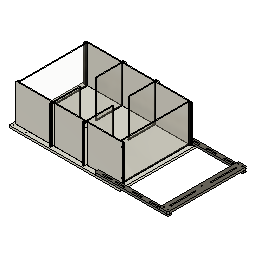
3ChamberBox (Autodesk Fusion 360 design; units mm, degrees)
Autodesk Fusion 360 part; units mm, degrees
sketch "Base" plane through (0, 0, 0) normal (0, 0, 1) x (1, 0, 0)
  line L0 (0, 0) -> (660.4, 0)
  line L1 (660.4, 0) -> (660.4, 469.9)
  line L2 (660.4, 469.9) -> (0, 469.9)
  line L3 (0, 469.9) -> (0, 0)
  line L4 (636.651, 437.261) -> (636.651, 32.639)
  line L5 (23.749, 32.639) -> (23.749, 437.261)
  line L6 (30.226, 32.639) -> (30.226, 437.261)
  line L7 (630.174, 437.261) -> (630.174, 32.639)
  line L8 (233.4895, 459.4352) -> (233.4895, 459.4352)
  line L9 (233.4895, 10.4648) -> (233.4895, 10.4648)
  line L10 (429.1965, 459.4352) -> (429.1965, 459.4352)
  line L11 (429.1965, 10.4648) -> (429.1965, 10.4648)
  line L12 (23.749, 437.261) -> (11.4935, 437.261)
  line L13 (8.255, 440.4995) -> (8.255, 440.4995)
  line L14 (11.4935, 443.738) -> (23.749, 443.738)
  line L15 (636.651, 437.261) -> (648.9065, 437.261)
  line L16 (652.145, 440.4995) -> (652.145, 440.4995)
  line L17 (648.9065, 443.738) -> (636.651, 443.738)
  line L18 (636.651, 26.162) -> (648.9065, 26.162)
  line L19 (652.145, 29.4005) -> (652.145, 29.4005)
  line L20 (648.9065, 32.639) -> (636.651, 32.639)
  line L21 (432.435, 13.7033) -> (432.435, 26.162)
  line L22 (432.435, 32.639) -> (432.435, 190.4057)
  line L23 (425.958, 190.4057) -> (425.958, 32.639)
  line L24 (425.958, 26.162) -> (425.958, 13.7033)
  line L25 (630.174, 32.639) -> (432.435, 32.639)
  line L26 (636.651, 26.162) -> (432.435, 26.162)
  line L27 (425.958, 32.639) -> (236.728, 32.639)
  line L28 (230.251, 32.639) -> (30.226, 32.639)
  line L29 (230.251, 13.7033) -> (230.251, 26.162)
  line L30 (230.251, 32.639) -> (230.251, 190.4057)
  line L31 (236.728, 190.4057) -> (236.728, 32.639)
  line L32 (236.728, 26.162) -> (236.728, 13.7033)
  line L33 (425.958, 26.162) -> (236.728, 26.162)
  line L34 (230.251, 26.162) -> (23.749, 26.162)
  line L35 (23.749, 443.738) -> (230.251, 443.738)
  line L36 (230.251, 282.6512) -> (230.251, 437.261)
  line L37 (230.251, 443.738) -> (230.251, 456.1967)
  line L38 (30.226, 437.261) -> (230.251, 437.261)
  line L39 (236.728, 456.1967) -> (236.728, 443.738)
  line L40 (236.728, 437.261) -> (236.728, 282.6512)
  line L41 (236.728, 443.738) -> (425.958, 443.738)
  line L42 (432.435, 443.738) -> (636.651, 443.738)
  line L43 (425.958, 456.1967) -> (425.958, 443.738)
  line L44 (425.958, 437.261) -> (425.958, 282.6512)
  line L45 (432.435, 282.6512) -> (432.435, 437.261)
  line L46 (432.435, 443.738) -> (432.435, 456.1967)
  line L47 (236.728, 437.261) -> (425.958, 437.261)
  line L48 (432.435, 437.261) -> (630.174, 437.261)
  line L49 (23.749, 26.162) -> (11.4935, 26.162)
  line L50 (8.255, 29.4005) -> (8.255, 29.4005)
  line L51 (11.4935, 32.639) -> (23.749, 32.639)
  arc A0 (8.255, 440.4995) -> (11.4935, 437.261) centre (11.4935, 440.4995) ccw
  arc A1 (11.4935, 443.738) -> (8.255, 440.4995) centre (11.4935, 440.4995) ccw
  arc A2 (233.4895, 459.4352) -> (230.251, 456.1967) centre (233.4895, 456.1967) ccw
  arc A3 (236.728, 456.1967) -> (233.4895, 459.4352) centre (233.4895, 456.1967) ccw
  arc A4 (429.1965, 459.4352) -> (425.958, 456.1967) centre (429.1965, 456.1967) ccw
  arc A5 (432.435, 456.1967) -> (429.1965, 459.4352) centre (429.1965, 456.1967) ccw
  arc A6 (652.145, 440.4995) -> (648.9065, 443.738) centre (648.9065, 440.4995) ccw
  arc A7 (648.9065, 437.261) -> (652.145, 440.4995) centre (648.9065, 440.4995) ccw
  arc A8 (652.145, 29.4005) -> (648.9065, 32.639) centre (648.9065, 29.4005) ccw
  arc A9 (648.9065, 26.162) -> (652.145, 29.4005) centre (648.9065, 29.4005) ccw
  arc A10 (429.1965, 10.4648) -> (432.435, 13.7033) centre (429.1965, 13.7033) ccw
  arc A11 (425.958, 13.7033) -> (429.1965, 10.4648) centre (429.1965, 13.7033) ccw
  arc A12 (230.251, 13.7033) -> (233.4895, 10.4648) centre (233.4895, 13.7033) ccw
  arc A13 (233.4895, 10.4648) -> (236.728, 13.7033) centre (233.4895, 13.7033) ccw
  arc A14 (8.255, 29.4005) -> (11.4935, 26.162) centre (11.4935, 29.4005) ccw
  arc A15 (11.4935, 32.639) -> (8.255, 29.4005) centre (11.4935, 29.4005) ccw
  line L52 (230.8352, 283.2354) -> (236.1438, 283.2354)
  line L53 (236.1438, 437.8452) -> (426.5422, 437.8452)
  line L54 (426.5422, 283.2354) -> (431.8508, 283.2354)
  line L55 (431.8508, 283.2354) -> (431.8508, 455.8538)
  line L56 (630.7582, 437.8452) -> (630.7582, 32.0548)
  line L57 (431.8508, 189.8215) -> (426.5422, 189.8215)
  line L58 (426.5422, 32.0548) -> (236.1438, 32.0548)
  line L59 (236.1438, 189.8215) -> (236.1438, 14.0462)
  line L60 (236.1438, 189.8215) -> (230.8352, 189.8215)
  line L61 (230.8352, 14.0462) -> (230.8352, 189.8215)
  line L62 (29.6418, 32.0548) -> (29.6418, 437.8452)
  line L63 (426.5422, 455.8538) -> (426.5422, 283.2354)
  line L64 (236.1438, 443.1538) -> (426.5422, 443.1538)
  line L65 (236.1438, 455.8538) -> (236.1438, 283.2354)
  line L66 (230.8352, 283.2354) -> (230.8352, 455.8538)
  line L67 (23.749, 443.1538) -> (230.8352, 443.1538)
  line L68 (11.6332, 443.1538) -> (23.749, 443.1538)
  line L69 (230.8352, 437.8452) -> (11.6332, 437.8452)
  line L70 (24.3332, 32.0548) -> (24.3332, 437.8452)
  line L71 (11.6332, 32.0548) -> (230.8352, 32.0548)
  line L72 (23.749, 26.7462) -> (11.6332, 26.7462)
  line L73 (230.8352, 26.7462) -> (23.749, 26.7462)
  line L74 (426.5422, 26.7462) -> (236.1438, 26.7462)
  line L75 (426.5422, 189.8215) -> (426.5422, 14.0462)
  line L76 (431.8508, 14.0462) -> (431.8508, 189.8215)
  line L77 (636.651, 26.7462) -> (431.8508, 26.7462)
  line L78 (636.651, 26.7462) -> (648.7668, 26.7462)
  line L79 (648.7668, 32.0548) -> (431.8508, 32.0548)
  line L80 (636.0668, 437.8452) -> (636.0668, 32.0548)
  line L81 (431.8508, 437.8452) -> (648.7668, 437.8452)
  line L82 (648.7668, 443.1538) -> (636.651, 443.1538)
  line L83 (431.8508, 443.1538) -> (636.651, 443.1538)
  line L84 (648.7668, 32.0548) -> (648.7668, 26.7462)
  line L85 (648.7668, 443.1538) -> (648.7668, 437.8452)
  line L86 (426.5422, 455.8538) -> (431.8508, 455.8538)
  line L87 (241.427, 455.8538) -> (230.8352, 455.8538)
  line L88 (11.6332, 437.8452) -> (11.6332, 443.1538)
  line L89 (11.6332, 32.0548) -> (11.6332, 26.7462)
  line L90 (230.8352, 14.0462) -> (236.1438, 14.0462)
  line L91 (421.259, 14.0462) -> (437.134, 14.0462)
  line L92 (437.134, 26.7462) -> (437.134, 14.0462)
  line L93 (421.259, 26.7462) -> (421.259, 14.0462)
  line L94 (241.427, 26.7462) -> (241.427, 14.0462)
  line L95 (241.427, 14.0462) -> (236.1438, 14.0462)
  line L96 (225.552, 26.7462) -> (225.552, 14.0462)
  line L97 (225.552, 14.0462) -> (230.8352, 14.0462)
  line L98 (11.6332, 32.0548) -> (11.6332, 37.338)
  line L99 (11.6332, 37.338) -> (24.3332, 37.338)
  line L100 (11.6332, 437.8452) -> (11.6332, 432.562)
  line L101 (11.6332, 432.562) -> (24.3332, 432.562)
  line L102 (225.552, 443.1538) -> (225.552, 455.8538)
  line L103 (225.552, 455.8538) -> (230.8352, 455.8538)
  line L104 (241.427, 443.1538) -> (241.427, 455.8538)
  line L105 (421.259, 443.1538) -> (421.259, 455.8538)
  line L106 (421.259, 455.8538) -> (426.5422, 455.8538)
  line L107 (437.134, 443.1538) -> (437.134, 455.8538)
  line L108 (437.134, 455.8538) -> (431.8508, 455.8538)
  line L109 (636.0668, 432.562) -> (648.7668, 432.562)
  line L110 (648.7668, 432.562) -> (648.7668, 437.8452)
  line L111 (636.0668, 37.338) -> (648.7668, 37.338)
  line L112 (648.7668, 37.338) -> (648.7668, 32.0548)
  circle A16 centre (12.7, 457.2) radius 2.5527
  circle A17 centre (88.9, 457.2) radius 2.5527
  circle A18 centre (12.7, 12.7) radius 2.5527
  circle A19 centre (88.9, 12.7) radius 2.5527
  circle A20 centre (647.7, 12.7) radius 2.5527
  circle A21 centre (571.5, 12.7) radius 2.5527
  circle A22 centre (647.7, 457.2) radius 2.5527
  circle A23 centre (571.5, 457.2) radius 2.5527
  arc A24 (236.728, 190.4057) -> (230.251, 190.4057) centre (233.4895, 190.4057) ccw
  arc A25 (230.251, 282.6512) -> (236.728, 282.6512) centre (233.4895, 282.6512) ccw
  arc A26 (425.958, 282.6512) -> (432.435, 282.6512) centre (429.1965, 282.6512) ccw
  arc A27 (432.435, 190.4057) -> (425.958, 190.4057) centre (429.1965, 190.4057) ccw
  dimension "d1" = 660.4
  dimension "d2" = 469.9
  dimension "d3" = 26.162
  dimension "d4" = 26.162
  dimension "d5" = 23.749
  dimension "d6" = 23.749
  dimension "d8" = 200.025
  dimension "d9" = 6.477
  dimension "d10" = 197.739
  dimension "d11" = 6.477
  dimension "d22" = 3.2385
  dimension "d30" = 12.7
  dimension "d31" = 12.7
  dimension "d33" = 12.7
  dimension "d34" = 5.2832
  dimension "d35" = 5.2832
  dimension "d36" = 5.2832
  dimension "d37" = 5.2832
  dimension "d38" = 12.7
  dimension "d39" = 12.7
  dimension "d40" = 12.7
  dimension "d41" = 12.7
  dimension "d42" = 5.2832
  dimension "d43" = 5.2832
  dimension "d44" = 12.7
  dimension "d45" = 12.7
  dimension "d46" = 12.7
  dimension "d47" = 190.3984
  dimension "d48" = 12.7
  dimension "d49" = 5.2832
  dimension "d50" = 5.2832
  dimension "d51" = 12.7
  dimension "d52" = 5.2832
  dimension "d53" = 12.7
  dimension "d54" = 12.7
  dimension "d55" = 5.2832
  dimension "d56" = 12.7
  dimension "d57" = 12.7
  dimension "d58" = 5.2832
  dimension "d59" = 12.7
  dimension "d60" = 5.2832
  dimension "d61" = 12.7
  dimension "d62" = 12.7
  dimension "d63" = 12.7
  dimension "d195" = 5.1054
  dimension "d196" = 5.1054
  dimension "d197" = 12.7
  dimension "d198" = 88.9
  dimension "d199" = 12.7
  dimension "d200" = 12.7
  dimension "d201" = 5.1054
  dimension "d202" = 5.1054
  dimension "d203" = 12.7
  dimension "d204" = 88.9
  dimension "d205" = 12.7
  dimension "d206" = 12.7
  dimension "d207" = 5.1054
  dimension "d208" = 5.1054
  dimension "d209" = 12.7
  dimension "d210" = 88.9
  dimension "d211" = 12.7
  dimension "d212" = 12.7
  dimension "d213" = 5.1054
  dimension "d214" = 5.1054
  dimension "d215" = 12.7
  dimension "d216" = 88.9
  dimension "d217" = 12.7
  dimension "d218" = 12.7
  constraint horizontal L0
  constraint vertical L1
  constraint horizontal L2
  constraint vertical L3
  constraint coincident L0.start L3.end
  constraint horizontal L35
  constraint vertical L4
  constraint horizontal L26
  constraint vertical L5
  constraint vertical L39
  constraint vertical L29
  constraint vertical L43
  constraint vertical L21
  constraint coincident L36.start L29
  constraint collinear L29 L36
  constraint collinear L31 L39
  constraint coincident L23.start L43
  constraint collinear L21 L45
  constraint collinear L23 L43
  constraint perpendicular L5 L12
  constraint perpendicular L5 L14
  constraint parallel L25 L26
  constraint parallel L5 L6
  constraint parallel L35 L38
  constraint parallel L4 L7
  constraint perpendicular L4 L15
  constraint perpendicular L4 L17
  constraint perpendicular L7 L18
  constraint perpendicular L4 L20
  constraint collinear L21 L22
  constraint coincident L23.end L25
  constraint coincident L24.start L26
  constraint collinear L23 L24
  constraint collinear L25 L27
  constraint collinear L26 L33
  constraint coincident L28.start L29
  constraint collinear L27 L28
  constraint coincident L29.end L33
  constraint collinear L29 L30
  constraint collinear L31 L32
  constraint collinear L33 L34
  constraint coincident L35.end L36
  constraint collinear L35 L41
  constraint collinear L36 L37
  constraint coincident L40.start L39
  constraint collinear L38 L47
  constraint collinear L39 L40
  constraint coincident L42.start L45
  constraint collinear L41 L42
  constraint collinear L43 L44
  constraint coincident L45.end L47
  constraint collinear L45 L46
  constraint collinear L47 L48
  constraint perpendicular L5 L49
  constraint perpendicular L5 L51
  constraint tangent L12 A0
  constraint tangent L14 A1
  constraint equal A0 A1
  constraint tangent L37 A2
  constraint equal A0 A2
  constraint tangent L39 A3
  constraint equal A0 A3
  constraint tangent L43 A4
  constraint equal A0 A4
  constraint tangent L46 A5
  constraint equal A0 A5
  constraint tangent L17 A6
  constraint equal A0 A6
  constraint tangent L15 A7
  constraint equal A0 A7
  constraint tangent L20 A8
  constraint equal A0 A8
  constraint tangent L18 A9
  constraint equal A0 A9
  constraint tangent L21 A10
  constraint equal A0 A10
  constraint tangent L24 A11
  constraint equal A0 A11
  constraint tangent L29 A12
  constraint equal A0 A12
  constraint tangent L32 A13
  constraint equal A0 A13
  constraint tangent L49 A14
  constraint equal A0 A14
  constraint tangent L51 A15
  constraint equal A0 A15
  constraint parallel L43 L63
  constraint parallel L41 L64
  constraint parallel L39 L65
  constraint parallel L37 L66
  constraint parallel L35 L67
  constraint parallel L14 L68
  constraint parallel L12 L69
  constraint parallel L5 L70
  constraint parallel L51 L71
  constraint parallel L49 L72
  constraint parallel L34 L73
  constraint parallel L29 L61
  constraint parallel L32 L59
  constraint parallel L33 L74
  constraint parallel L24 L75
  constraint parallel L21 L76
  constraint parallel L26 L77
  constraint parallel L18 L78
  constraint parallel L20 L79
  constraint parallel L4 L80
  constraint parallel L15 L81
  constraint parallel L17 L82
  constraint parallel L42 L83
  constraint parallel L46 L55
  constraint coincident L67.end L66
  constraint parallel L40 L65
  constraint parallel L47 L53
  constraint parallel L44 L63
  constraint parallel L45 L55
  constraint parallel L48 L81
  constraint parallel L7 L56
  constraint parallel L25 L79
  constraint parallel L22 L76
  constraint parallel L23 L75
  constraint parallel L27 L58
  constraint parallel L31 L59
  constraint parallel L30 L61
  constraint parallel L28 L71
  constraint parallel L6 L62
  constraint parallel L38 L69
  constraint parallel L36 L66
  constraint coincident L64.start L65
  constraint coincident L64.end L63
  constraint coincident L81.start L55
  constraint coincident L77.end L76
  constraint coincident L74.start L75
  constraint coincident L71.end L61
  constraint coincident L58.end L59
  constraint perpendicular L78 L84
  constraint perpendicular L82 L85
  constraint perpendicular L55 L86
  constraint perpendicular L65 L87
  constraint perpendicular L68 L88
  constraint perpendicular L72 L89
  constraint perpendicular L61 L90
  constraint perpendicular L76 L91
  constraint coincident L77 L92.start
  constraint perpendicular L26 L92
  constraint perpendicular L21 L91
  constraint coincident L74 L93.start
  constraint perpendicular L33 L93
  constraint perpendicular L24 L91
  constraint coincident L74 L94.start
  constraint perpendicular L33 L94
  constraint coincident L59 L90.end
  constraint perpendicular L59 L95
  constraint coincident L73 L96.start
  constraint perpendicular L34 L96
  constraint coincident L61 L90.start
  constraint perpendicular L61 L97
  constraint coincident L71 L89.start
  constraint perpendicular L51 L98
  constraint coincident L70 L99.end
  constraint perpendicular L70 L99
  constraint coincident L69 L88.start
  constraint perpendicular L12 L100
  constraint coincident L70 L101.end
  constraint perpendicular L70 L101
  constraint coincident L67 L102.start
  constraint perpendicular L67 L102
  constraint coincident L66 L87.end
  constraint perpendicular L66 L103
  constraint coincident L64 L104.start
  constraint perpendicular L41 L104
  constraint perpendicular L39 L87
  constraint coincident L64 L105.start
  constraint perpendicular L64 L105
  constraint coincident L63 L86.start
  constraint perpendicular L63 L106
  constraint coincident L83 L107.start
  constraint perpendicular L42 L107
  constraint coincident L55 L86.end
  constraint perpendicular L55 L108
  constraint coincident L80 L109.start
  constraint perpendicular L80 L109
  constraint coincident L81 L85.end
  constraint perpendicular L81 L110
  constraint coincident L80 L111.start
  constraint perpendicular L80 L111
  constraint coincident L79 L84.start
  constraint perpendicular L79 L112
  constraint tangent L40 A25
  constraint tangent L31 A24
  constraint tangent L45 A26
  constraint tangent L22 A27
  measures "d1" distance of L0.start L0.end
  measures "d2" distance of L0.start L2.end
  measures "d3" distance of L2 L35
  measures "d4" distance of L0 L26
  measures "d5" distance of L3 L5
  measures "d6" distance of L1 L4
  measures "d8" distance of L6 L29
  measures "d9" distance of L29 L39
  measures "d10" distance of L7 L21
  measures "d11" distance of L21 L43
  measures "d22" radius of A0
  measures "d30" distance of L77 L91
  measures "d31" distance of L74 L91
  measures "d33" distance of L74 L91
  measures "d34" distance of L76 L92
  measures "d35" distance of L75 L93
  measures "d36" distance of L61 L96
  measures "d37" distance of L59 L94
  measures "d38" distance of L73 L97
  measures "d39" distance of L73 L90
  measures "d40" distance of L74 L95
  measures "d41" distance of L70 L98
  measures "d42" distance of L71 L99
  measures "d43" distance of L69 L101
  measures "d44" distance of L70 L100
  measures "d45" distance of L67 L103
  measures "d46" distance of L67 L87
  measures "d47" distance of L64.end L64.start
  measures "d48" distance of L64 L87
  measures "d49" distance of L65 L104
  measures "d50" distance of L66 L102
  measures "d51" distance of L64 L106
  measures "d52" distance of L63 L105
  measures "d53" distance of L64 L86
  measures "d54" distance of L83 L108
  measures "d55" distance of L55 L107
  measures "d56" distance of L80 L110
  measures "d57" distance of L80 L85
  measures "d58" distance of L81 L109
  measures "d59" distance of L80 L112
  measures "d60" distance of L79 L111
  measures "d61" distance of L80 L84
  measures "d62" distance of L70 L88
  measures "d63" distance of L70 L89
  measures "d195" diameter of A16
  measures "d196" diameter of A17
  measures "d197" distance of L3 A16.centre
  measures "d198" distance of L3 A17.centre
  measures "d199" distance of L2 A16.centre
  measures "d200" distance of L2 A17.centre
  measures "d201" diameter of A18
  measures "d202" diameter of A19
  measures "d203" distance of L3 A18.centre
  measures "d204" distance of L3 A19.centre
  measures "d205" distance of L0 A18.centre
  measures "d206" distance of L0 A19.centre
  measures "d207" diameter of A20
  measures "d208" diameter of A21
  measures "d209" distance of L1 A20.centre
  measures "d210" distance of L1 A21.centre
  measures "d211" distance of L0 A20.centre
  measures "d212" distance of L0 A21.centre
  measures "d213" diameter of A22
  measures "d214" diameter of A23
  measures "d215" distance of L1 A22.centre
  measures "d216" distance of L1 A23.centre
  measures "d217" distance of L2 A22.centre
  measures "d218" distance of L2 A23.centre
extrude "Extrude1" add sketch "Base" against normal blind 12.7 contours L0 L1 L2 L3 | L4 L15 L109 L110 | L4 L15 L80 L81 L109 L110 | L4 L80 L109 L111 | L15 L17 L42 A6 A7 L82 L83 L85 L107 L110 | L4 L20 L111 L112 | L4 L20 L79 L80 L111 L112 | L56 L79 L80 L81 | L55 L81 L82 L83 L85 | L18 L20 L26 A8 A9 L77 L78 L84 L92 L112 | L76 L77 L78 L79 L84 | L52 L53 L54 L55 L56 L57 L58 L59 L60 L61 L62 L63 L65 L66 L69 L71 L75 L76 L79 L81 | L54 L55 L63 L86 | L42 L46 L55 L83 L107 L108 | L57 L75 L76 L91 | L42 L46 L107 L108 | L21 L26 L76 L77 L91 L92 | L43 L46 A4 A5 L86 L106 L108 | L21 L24 A10 A11 L91 | L53 L63 L64 L65 | L41 L43 L63 L64 L105 L106 | L21 L26 L91 L92 | L24 L33 L74 L75 L91 L93 | L58 L59 L74 L75 | L52 L65 L66 L87 | L41 L43 L105 L106 | L24 L33 L91 L93 | L59 L60 L61 L90 | L39 L41 L64 L65 L87 L104 | L41 L64 L104 L105 | L33 L74 L93 L94 | L32 L33 L59 L74 L94 L95 | L37 L39 A2 A3 L87 L103 | L29 L32 A12 A13 L90 L95 L97 | L39 L41 L87 L104 | L35 L37 L66 L67 L102 L103 | L66 L67 L68 L69 L88 | L32 L33 L94 L95 | L61 L71 L72 L73 L89 | L29 L34 L61 L73 L96 L97 | L35 L37 L102 L103 | L62 L69 L70 L71 | L29 L34 L96 L97 | L12 L14 L35 A0 A1 L67 L68 L88 L100 L102 | L5 L12 L69 L70 L100 L101 | L34 L49 L51 A14 A15 L72 L73 L89 L96 L98 | L5 L51 L70 L71 L98 L99 | L5 L70 L99 L101 | L5 L12 L100 L101 | L5 L51 L98 L99 | L6 L7 L22 L23 L25 L27 L28 L30 L31 L36 L38 L40 L44 L45 L47 L48 A24 A25 A26 A27 | A16 | A17 | A18 | A19 | A20 | A21 | A22 | A23 makes body 1
extrude "Extrude2" cut sketch "Base" against normal blind 3.3528 contours L4 L15 L80 L81 L109 L110 | L4 L80 L109 L111 | L15 L17 L42 A6 A7 L82 L83 L85 L107 L110 | L4 L20 L79 L80 L111 L112 | L56 L79 L80 L81 | L55 L81 L82 L83 L85 | L18 L20 L26 A8 A9 L77 L78 L84 L92 L112 | L76 L77 L78 L79 L84 | L52 L53 L54 L55 L56 L57 L58 L59 L60 L61 L62 L63 L65 L66 L69 L71 L75 L76 L79 L81 | L54 L55 L63 L86 | L42 L46 L55 L83 L107 L108 | L57 L75 L76 L91 | L21 L26 L76 L77 L91 L92 | L43 L46 A4 A5 L86 L106 L108 | L21 L24 A10 A11 L91 | L53 L63 L64 L65 | L41 L43 L63 L64 L105 L106 | L24 L33 L74 L75 L91 L93 | L58 L59 L74 L75 | L52 L65 L66 L87 | L59 L60 L61 L90 | L39 L41 L64 L65 L87 L104 | L41 L64 L104 L105 | L33 L74 L93 L94 | L32 L33 L59 L74 L94 L95 | L37 L39 A2 A3 L87 L103 | L29 L32 A12 A13 L90 L95 L97 | L35 L37 L66 L67 L102 L103 | L66 L67 L68 L69 L88 | L61 L71 L72 L73 L89 | L29 L34 L61 L73 L96 L97 | L62 L69 L70 L71 | L12 L14 L35 A0 A1 L67 L68 L88 L100 L102 | L5 L12 L69 L70 L100 L101 | L34 L49 L51 A14 A15 L72 L73 L89 L96 L98 | L5 L51 L70 L71 L98 L99 | L5 L70 L99 L101 bodies 1
extrude "Extrude3" add sketch "Base" along normal blind 220.8022 separate body contours L54 L55 L63 L86 | L57 L75 L76 L91 | L52 L65 L66 L87 | L59 L60 L61 L90 makes body 2 at (431.8508, 340.7749, 73.6007) makes body 3 at (431.8508, 72.638, 147.2015) makes body 4 at (236.1438, 398.3143, 73.6007) makes body 5 at (236.1438, 131.2297, 73.6007)
extrude "Extrude4" add sketch "Base" along normal blind 220.8022 separate body contours L56 L79 L80 L81 | L62 L69 L70 L71 makes body 6 at (29.6418, 167.3183, 73.6007) makes body 7 at (636.0668, 302.5817, 73.6007)
extrude "Extrude5" add sketch "Base" along normal blind 220.8022 separate body contours L4 L20 L111 L112 | L4 L20 L79 L80 L111 L112 makes body 8
extrude "Extrude6" add sketch "Base" along normal blind 220.8022 separate body contours L4 L15 L109 L110 | L4 L15 L80 L81 L109 L110 makes body 9
extrude "Extrude7" add sketch "Base" along normal blind 220.8022 separate body contours L42 L46 L55 L83 L107 L108 | L42 L46 L107 L108 | L41 L43 L63 L64 L105 L106 | L41 L43 L105 L106 makes body 10 at (437.134, 447.3871, 147.2015) makes body 11 at (426.5422, 451.6205, 147.2015)
extrude "Extrude8" add sketch "Base" along normal blind 220.8022 separate body contours L21 L26 L76 L77 L91 L92 | L21 L26 L91 L92 | L24 L33 L74 L75 L91 L93 | L24 L33 L91 L93 makes body 12 at (437.134, 22.5129, 147.2015) makes body 13 at (421.259, 22.5129, 147.2015)
extrude "Extrude9" add sketch "Base" along normal blind 220.8022 separate body contours L32 L33 L59 L74 L94 L95 | L32 L33 L94 L95 | L29 L34 L61 L73 L96 L97 | L29 L34 L96 L97 makes body 14 at (236.1438, 22.5129, 73.6007) makes body 15 at (225.552, 22.5129, 147.2015)
extrude "Extrude10" add sketch "Base" along normal blind 220.8022 separate body contours L39 L41 L64 L65 L87 L104 | L39 L41 L87 L104 | L35 L37 L66 L67 L102 L103 | L35 L37 L102 L103 makes body 16 at (236.1438, 451.6205, 147.2015) makes body 17 at (230.8352, 447.3871, 147.2015)
extrude "Extrude11" add sketch "Base" along normal blind 220.8022 separate body contours L5 L12 L69 L70 L100 L101 | L5 L12 L100 L101 makes body 18
extrude "Extrude12" add sketch "Base" along normal blind 220.8022 separate body contours L5 L51 L70 L71 L98 L99 | L5 L51 L98 L99 makes body 19
extrude "Extrude13" add sketch "Base" along normal blind 224.155 separate body contours L55 L81 L82 L83 L85 | L76 L77 L78 L79 L84 | L53 L63 L64 L65 | L58 L59 L74 L75 | L66 L67 L68 L69 L88 | L61 L71 L72 L73 L89 makes body 20 at (504.1561, 443.1538, 74.7183) makes body 21 at (157.7679, 26.7462, 74.7183) makes body 22 at (299.6099, 437.8452, 149.4367) makes body 23 at (504.1561, 26.7462, 74.7183) makes body 24 at (363.0761, 26.7462, 149.4367) makes body 25 at (84.7005, 437.8452, 149.4367)
extrude "Extrude14" cut 12 faces at (435.3729, 22.5129, 0) (423.0201, 18.2795, 0) (237.9049, 18.2795, 0) (227.3131, 18.2795, 0) (19.9051, 34.0106, 0) (19.9051, 435.8894, 0) (229.0741, 447.3871, 0) (237.9049, 451.6205, 0) (435.3729, 447.3871, 0) (423.0201, 451.6205, 0) (640.4949, 435.8894, 0) (640.4949, 34.0106, 0) along direction (0, 0, 1) blind 1.7272 on bodies 8 9 10 11 12 13 14 15 16 17 18 19 bodies 8 9 10 11 13 12 14 15 16 17 18 19
extrude "Extrude15" add 6 faces at (157.7679, 28.5157, 0) (363.0761, 28.5157, 0) (576.4615, 30.2853, 0) (576.4615, 441.3843, 0) (363.0761, 439.6147, 0) (84.7005, 441.3843, 0) along direction (0, 0, -1) blind 3.3528 on bodies 20 21 22 23 24 25 bodies 21 20 22 23 24 25
extrude "Extrude16" add 6 faces at (632.5277, 302.5817, 0) (428.3117, 398.3143, 0) (428.3117, 131.2297, 0) (232.6047, 398.3143, 0) (232.6047, 131.2297, 0) (26.1027, 302.5817, 0) along direction (0, 0, -1) blind 3.3528 on bodies 2 3 4 5 6 7 bodies 7 2 3 4 5 6
extrude "Extrude17" cut 6 faces at (576.4615, 30.2853, 224.155) (363.0761, 28.5157, 224.155) (157.7679, 30.2853, 224.155) (576.4615, 441.3843, 224.155) (363.0761, 439.6147, 224.155) (84.7005, 441.3843, 224.155) along direction (0, 0, -1) blind 3.3528 on bodies 20 21 22 23 24 25 bodies 20 21 22 23 24 25
fillet "Fillet1" radius 6.35 20 edges at (429.1965, 455.8538, 220.8022) (429.1965, 14.0462, 220.8022) (233.4895, 455.8538, 220.8022) (233.4895, 14.0462, 220.8022) (648.7668, 34.6964, 220.8022) (648.7668, 435.2036, 220.8022) (434.4924, 455.8538, 220.8022) (423.9006, 455.8538, 220.8022) (434.4924, 14.0462, 220.8022) (423.9006, 14.0462, 220.8022) (238.7854, 14.0462, 220.8022) (228.1936, 14.0462, 220.8022) (238.7854, 455.8538, 220.8022) (228.1936, 455.8538, 220.8022) (11.6332, 435.2036, 220.8022) (11.6332, 34.6964, 220.8022) (648.7668, 440.4995, 220.8022) (11.6332, 29.4005, 220.8022) (648.7668, 29.4005, 220.8022) (11.6332, 440.4995, 220.8022) on bodies 2 3 4 5 8 9 10 11 12 13 14 15 16 17 18 19 20 21 23 25
sketch "Small Wall Tapped" plane through (437.134, 0, 0) normal (1, 0, 0) x (0, 1, 0)
  arc A0 (20.3962, 220.8022) -> (14.0462, 214.4522) centre (20.3962, 214.4522) ccw
  line L0 (14.0462, 214.4522) -> (14.0462, 1.7272)
  line L1 (14.0462, 1.7272) -> (26.7462, 1.7272)
  line L2 (26.7462, 1.7272) -> (26.7462, 220.8022)
  line L3 (26.7462, 220.8022) -> (20.3962, 220.8022)
  circle A1 centre (20.3962, 34.1122) radius 1.3525
  circle A2 centre (20.3962, 195.4022) radius 1.3526
  dimension "d96" = 2.7051
  dimension "d97" = 32.385
  dimension "d98" = 2.7051
  dimension "d99" = 25.4
  measures "d96" diameter of A1
  measures "d97" distance of L1 A1.centre
  measures "d98" diameter of A2
  measures "d99" distance of L3 A2.centre
extrude "Extrude18" cut sketch "Small Wall Tapped" against normal up to surface (15.875 mm away) contours A1 | A2 bodies 12
thread "Thread1" "ANSI Unified Screw Threads 0.138(#6) 6-32 UNC 3B" major diameter 3.5052 minor diameter 2.7686 pitch 0.7937 angle 60 resizes the face on face at (435.3729, 21.0132, 196.6058) on bodies 12
thread "Thread2" "ANSI Unified Screw Threads 0.138(#6) 6-32 UNC 3B" major diameter 3.5052 minor diameter 2.7686 pitch 0.7937 angle 60 resizes the face on face at (433.6119, 21.4744, 34.9289) on bodies 12
sketch "Camera Sled" plane through (0, 0, 0) normal (0, 0, 1) x (1, 0, 0)
  line L0 (514.35, 0) -> (939.165, 0)
  circle A0 centre (647.7, 12.7) radius 2.5527
  circle A1 centre (571.5, 12.7) radius 2.5527
  circle A2 centre (647.7, 457.2) radius 2.5527
  circle A3 centre (571.5, 457.2) radius 2.5527
  line L1 (514.35, 469.9) -> (939.165, 469.9)
  line L2 (406.4, 0) -> (660.4, 0)
  line L3 (660.4, 0) -> (660.4, 469.9)
  line L4 (660.4, 469.9) -> (406.4, 469.9)
  line L5 (406.4, 443.738) -> (425.958, 443.738)
  line L6 (425.958, 443.738) -> (425.958, 456.1967)
  arc A4 (432.435, 456.1967) -> (425.958, 456.1967) centre (429.1965, 456.1967) ccw
  line L7 (432.435, 456.1967) -> (432.435, 443.738)
  line L8 (432.435, 443.738) -> (648.9065, 443.738)
  arc A5 (648.9065, 437.261) -> (648.9065, 443.738) centre (648.9065, 440.4995) ccw
  line L9 (648.9065, 437.261) -> (636.651, 437.261)
  line L10 (636.651, 437.261) -> (636.651, 32.639)
  line L11 (636.651, 32.639) -> (648.9065, 32.639)
  arc A6 (648.9065, 26.162) -> (648.9065, 32.639) centre (648.9065, 29.4005) ccw
  line L12 (648.9065, 26.162) -> (432.435, 26.162)
  line L13 (432.435, 26.162) -> (432.435, 13.7033)
  arc A7 (425.958, 13.7033) -> (432.435, 13.7033) centre (429.1965, 13.7033) ccw
  line L14 (425.958, 13.7033) -> (425.958, 26.162)
  line L15 (425.958, 26.162) -> (406.4, 26.162)
  line L16 (425.958, 437.261) -> (406.4, 437.261)
  line L17 (406.4, 32.639) -> (425.958, 32.639)
  line L18 (425.958, 32.639) -> (425.958, 190.4057)
  line L19 (425.958, 190.4057) -> (432.435, 190.4057)
  line L20 (432.435, 190.4057) -> (432.435, 32.639)
  line L21 (432.435, 32.639) -> (630.174, 32.639)
  line L22 (630.174, 32.639) -> (630.174, 437.261)
  line L23 (630.174, 437.261) -> (432.435, 437.261)
  line L24 (432.435, 437.261) -> (432.435, 282.6512)
  line L25 (432.435, 282.6512) -> (425.958, 282.6512)
  line L26 (425.958, 282.6512) -> (425.958, 437.261)
  line L27 (894.715, 25.4) -> (894.715, 444.5)
  line L28 (945.515, 25.4) -> (945.515, 444.5)
  line L29 (945.515, 25.4) -> (945.515, 6.35)
  line L30 (945.515, 444.5) -> (945.515, 463.55)
  line L31 (508, 6.35) -> (508, 19.05)
  line L32 (508, 463.55) -> (508, 450.85)
  circle A8 centre (910.6535, 234.95) radius 3.2385
  line L33 (894.715, 25.4) -> (894.715, 0)
  line L34 (894.715, 444.5) -> (894.715, 469.9)
  line L35 (546.1, 460.502) -> (596.9, 460.502)
  line L36 (622.3, 460.502) -> (673.1, 460.502)
  line L37 (546.1, 453.898) -> (596.9, 453.898)
  line L38 (622.3, 453.898) -> (673.1, 453.898)
  arc A9 (596.9, 453.898) -> (596.9, 460.502) centre (596.9, 457.2) ccw
  arc A10 (546.1, 460.502) -> (546.1, 453.898) centre (546.1, 457.2) ccw
  arc A11 (622.3, 460.502) -> (622.3, 453.898) centre (622.3, 457.2) ccw
  arc A12 (673.1, 453.898) -> (673.1, 460.502) centre (673.1, 457.2) ccw
  line L39 (546.1, 9.398) -> (596.9, 9.398)
  line L40 (622.3, 9.398) -> (673.1, 9.398)
  line L41 (546.1, 16.002) -> (596.9, 16.002)
  line L42 (622.3, 16.002) -> (673.1, 16.002)
  arc A13 (596.9, 9.398) -> (596.9, 16.002) centre (596.9, 12.7) ccw
  arc A14 (546.1, 16.002) -> (546.1, 9.398) centre (546.1, 12.7) ccw
  arc A15 (622.3, 16.002) -> (622.3, 9.398) centre (622.3, 12.7) ccw
  arc A16 (673.1, 9.398) -> (673.1, 16.002) centre (673.1, 12.7) ccw
  circle A17 centre (907.415, 12.7) radius 2.5527
  circle A18 centre (932.815, 12.7) radius 2.5527
  circle A19 centre (907.415, 457.2) radius 2.5527
  circle A20 centre (932.815, 457.2) radius 2.5527
  circle A21 centre (907.415, 12.7) radius 3.302
  circle A22 centre (932.815, 12.7) radius 3.302
  circle A23 centre (907.415, 457.2) radius 3.302
  circle A24 centre (932.815, 457.2) radius 3.302
  line L43 (808.355, 279.4) -> (808.355, 279.4)
  line L44 (923.417, 282.702) -> (923.417, 428.498)
  line L45 (808.355, 431.8) -> (808.355, 431.8)
  line L46 (916.813, 428.498) -> (916.813, 282.702)
  line L47 (808.355, 190.5) -> (808.355, 190.5)
  line L48 (923.417, 187.198) -> (923.417, 41.402)
  line L49 (808.355, 38.1) -> (808.355, 38.1)
  line L50 (916.813, 41.402) -> (916.813, 187.198)
  arc A25 (916.813, 41.402) -> (920.115, 38.1) centre (920.115, 41.402) ccw
  arc A26 (920.115, 38.1) -> (923.417, 41.402) centre (920.115, 41.402) ccw
  arc A27 (920.115, 190.5) -> (916.813, 187.198) centre (920.115, 187.198) ccw
  arc A28 (923.417, 187.198) -> (920.115, 190.5) centre (920.115, 187.198) ccw
  arc A29 (916.813, 282.702) -> (920.115, 279.4) centre (920.115, 282.702) ccw
  arc A30 (920.115, 279.4) -> (923.417, 282.702) centre (920.115, 282.702) ccw
  arc A31 (920.115, 431.8) -> (916.813, 428.498) centre (920.115, 428.498) ccw
  arc A32 (923.417, 428.498) -> (920.115, 431.8) centre (920.115, 428.498) ccw
  line L51 (514.35, 25.4) -> (945.515, 25.4)
  line L52 (945.515, 444.5) -> (514.35, 444.5)
  line L53 (406.4, 0) -> (406.4, 469.9)
  arc A33 (508, 6.35) -> (514.35, 0) centre (514.35, 6.35) ccw
  arc A34 (514.35, 25.4) -> (508, 19.05) centre (514.35, 19.05) ccw
  arc A35 (514.35, 469.9) -> (508, 463.55) centre (514.35, 463.55) ccw
  arc A36 (508, 450.85) -> (514.35, 444.5) centre (514.35, 450.85) ccw
  arc A37 (945.515, 463.55) -> (939.165, 469.9) centre (939.165, 463.55) ccw
  arc A38 (939.165, 0) -> (945.515, 6.35) centre (939.165, 6.35) ccw
  line L54 (622.3, 16.002) -> (673.1, 16.002)
  arc A39 (622.3, 16.002) -> (622.3, 9.398) centre (622.3, 12.7) ccw
  line L55 (622.3, 9.398) -> (673.1, 9.398)
  arc A40 (673.1, 9.398) -> (673.1, 16.002) centre (673.1, 12.7) ccw
  line L56 (723.9, 9.398) -> (774.7, 9.398)
  arc A41 (723.9, 16.002) -> (723.9, 9.398) centre (723.9, 12.7) ccw
  line L57 (723.9, 16.002) -> (774.7, 16.002)
  arc A42 (774.7, 9.398) -> (774.7, 16.002) centre (774.7, 12.7) ccw
  line L58 (723.9, 460.502) -> (774.7, 460.502)
  arc A43 (723.9, 460.502) -> (723.9, 453.898) centre (723.9, 457.2) ccw
  line L59 (723.9, 453.898) -> (774.7, 453.898)
  arc A44 (774.7, 453.898) -> (774.7, 460.502) centre (774.7, 457.2) ccw
  line L60 (825.5, 9.398) -> (876.3, 9.398)
  arc A45 (825.5, 16.002) -> (825.5, 9.398) centre (825.5, 12.7) ccw
  line L61 (825.5, 16.002) -> (876.3, 16.002)
  arc A46 (876.3, 9.398) -> (876.3, 16.002) centre (876.3, 12.7) ccw
  line L62 (825.5, 460.502) -> (876.3, 460.502)
  arc A47 (825.5, 460.502) -> (825.5, 453.898) centre (825.5, 457.2) ccw
  line L63 (825.5, 453.898) -> (876.3, 453.898)
  arc A48 (876.3, 453.898) -> (876.3, 460.502) centre (876.3, 457.2) ccw
  point P0 (916.813, 279.4)
  point P1 (923.417, 279.4)
  point P2 (916.813, 431.8)
  point P3 (916.813, 190.5)
  point P4 (923.417, 190.5)
  point P5 (916.813, 38.1)
  dimension "d102" = 5.1054
  dimension "d103" = 5.1054
  dimension "d105" = 76.2
  dimension "d106" = 5.1054
  dimension "d107" = 5.1054
  dimension "d111" = 462.28
  dimension "d112" = 50.8
  dimension "d116" = 152.4
  dimension "d117" = 152.4
  dimension "d118" = 6.477
  dimension "d119" = 15.9385
  dimension "d123" = 6.604
  dimension "d124" = 6.604
  dimension "d125" = 25.4
  dimension "d126" = 25.4
  dimension "d127" = 6.604
  dimension "d128" = 25.4
  dimension "d129" = 6.604
  dimension "d130" = 25.4
  dimension "d131" = 6.604
  dimension "d132" = 6.604
  dimension "d133" = 6.604
  dimension "d134" = 6.604
  dimension "d135" = 25.4
  dimension "d136" = 25.4
  dimension "d137" = 25.4
  dimension "d138" = 25.4
  dimension "d145" = 5.1054
  dimension "d146" = 5.1054
  dimension "d147" = 12.7
  dimension "d148" = 12.7
  dimension "d149" = 12.7
  dimension "d150" = 12.7
  dimension "d151" = 5.1054
  dimension "d152" = 5.1054
  dimension "d153" = 12.7
  dimension "d154" = 12.7
  dimension "d155" = 12.7
  dimension "d156" = 12.7
  dimension "d157" = 6.604
  dimension "d158" = 6.604
  dimension "d159" = 6.604
  dimension "d160" = 6.604
  dimension "d165" = 6.604
  dimension "d166" = 152.4
  dimension "d168" = 6.604
  dimension "d169" = 152.4
  dimension "d171" = 22.098
  dimension "d172" = 22.098
  dimension "d173" = 3.302
  dimension "d177" = 6.35
  dimension "d180" = 6.35
  dimension "d185" = 6.604
  dimension "d186" = 6.604
  dimension "d189" = 101.6
  dimension "d190" = 0
  constraint horizontal L0
  constraint coincident L27.end L52
  constraint perpendicular L27 L52
  constraint perpendicular L28 L52
  constraint perpendicular L0 L29
  constraint perpendicular L1 L30
  constraint perpendicular L32 L52
  constraint coincident L0 L33.end
  constraint perpendicular L0 L33
  constraint coincident L1 L34.end
  constraint perpendicular L1 L34
  constraint tangent L37 A12
  constraint perpendicular L3 L37
  constraint tangent L35 A12
  constraint collinear L35 L36
  constraint collinear L37 L38
  constraint tangent L41 A16
  constraint tangent L39 A16
  constraint perpendicular L3 L39
  constraint collinear L39 L40
  constraint collinear L41 L42
  constraint concentric A17 A21
  constraint concentric A18 A22
  constraint concentric A19 A23
  constraint concentric A20 A24
  constraint vertical L44
  constraint vertical L46
  constraint vertical L48
  constraint vertical L50
  constraint coincident P5 L50
  constraint tangent L50 A25
  constraint tangent L48 A26
  constraint equal A25 A26
  constraint coincident P3 L50
  constraint tangent L50 A27
  constraint equal A25 A27
  constraint coincident P4 L47
  constraint coincident P4 L48
  constraint tangent L48 A28
  constraint equal A25 A28
  constraint coincident P0 L46
  constraint tangent L46 A29
  constraint equal A25 A29
  constraint coincident P1 L43
  constraint coincident P1 L44
  constraint tangent L44 A30
  constraint equal A25 A30
  constraint coincident P2 L46
  constraint tangent L46 A31
  constraint equal A25 A31
  constraint tangent L44 A32
  constraint equal A25 A32
  constraint perpendicular L16 L53
  constraint coincident L53 L15.end
  constraint coincident L53 L17.start
  constraint coincident L53 L16.end
  constraint coincident L53 L5.start
  constraint tangent L31 A33
  constraint tangent L0 A33
  constraint tangent L31 A34
  constraint tangent L51 A34
  constraint equal A33 A34
  constraint tangent L32 A35
  constraint tangent L1 A35
  constraint equal A33 A35
  constraint tangent L32 A36
  constraint tangent L52 A36
  constraint equal A33 A36
  constraint tangent L30 A37
  constraint tangent L1 A37
  constraint equal A33 A37
  constraint tangent L29 A38
  constraint tangent L0 A38
  measures "d102" diameter of A0
  measures "d103" diameter of A1
  measures "d105" distance of A0.centre A1.centre
  measures "d106" diameter of A2
  measures "d107" diameter of A3
  measures "d111" distance of L20 L27
  measures "d112" distance of L27 L28
  measures "d116" distance of L3 L31
  measures "d117" distance of L3 L32
  measures "d118" diameter of A8
  measures "d119" distance of L27 A8.centre
  measures "d123" diameter of A10
  measures "d124" diameter of A12
  measures "d125" distance of A2.centre A12.centre
  measures "d126" distance of A3.centre A10.centre
  measures "d127" diameter of A9
  measures "d128" distance of A3.centre A9.centre
  measures "d129" diameter of A11
  measures "d130" distance of A2.centre A11.centre
  measures "d131" diameter of A14
  measures "d132" diameter of A13
  measures "d133" diameter of A15
  measures "d134" diameter of A16
  measures "d135" distance of A0.centre A16.centre
  measures "d136" distance of A0.centre A15.centre
  measures "d137" distance of A1.centre A13.centre
  measures "d138" distance of A1.centre A14.centre
  measures "d145" diameter of A17
  measures "d146" diameter of A18
  measures "d147" distance of L29 A18.centre
  measures "d148" distance of L33 A17.centre
  measures "d149" distance of L0 A17.centre
  measures "d150" distance of L0 A18.centre
  measures "d151" diameter of A19
  measures "d152" diameter of A20
  measures "d153" distance of L30 A20.centre
  measures "d154" distance of L34 A19.centre
  measures "d155" distance of A19.centre L52
  measures "d156" distance of A20.centre L52
  measures "d157" diameter of A21
  measures "d158" diameter of A22
  measures "d159" diameter of A23
  measures "d160" diameter of A24
  measures "d165" distance of P0 P1
  measures "d166" distance of P0 P2
  measures "d168" distance of P3 P4
  measures "d169" distance of P3 P5
  measures "d171" distance of L28 L48
  measures "d172" distance of L28 L44
  measures "d173" radius of A25
  measures "d177" radius of A33
  measures "d180" radius of A38
  measures "d185" diameter of A39
  measures "d186" diameter of A40
extrude "Extrude19" cut sketch "Camera Sled" against normal up to surface (12.7 mm away) contours A0 | A1 | A2 | A3 bodies 1
extrude "Extrude25" add sketch "Camera Sled" along normal blind 12.192 separate body contours L0 L2 L3 L31 L40 L42 A15 L51 A33 A34 L54 A39 L55 | L0 L3 L33 L40 L42 A16 L51 L54 L55 A40 | L0 L29 L33 L51 A38 | L1 L3 L34 L36 L38 A12 L52 | L1 L30 L34 L52 A37 | L1 L3 L4 L32 L36 L38 A11 L52 A35 A36 | A21 | A22 | A23 | A24 makes body 26 at (523.8327, 12.7, 0) makes body 27 at (523.8327, 457.2, 12.192)
extrude "Extrude26" add sketch "Camera Sled" along normal blind 12.7 separate body contours L0 L29 L33 L51 A38 | L27 L28 L51 L52 | L1 L30 L34 L52 A37 makes body 28
move_body "Move2" bodies 28 to x (1, 0, 0) y (0, 1, 0) z (0, 0, 1) at (0, 0, 12.192)
fillet "Fillet3" radius 6.35 2 edges at (945.515, 25.4, 6.096) (945.515, 444.5, 6.096) on bodies 26 27
sketch "Small Wall Thru Hole" plane through (421.259, 0, 0) normal (-1, 0, 0) x (0, -1, 0)
  circle A0 centre (-20.3962, 195.4022) radius 1.3843
  circle A1 centre (-20.3962, 34.1122) radius 1.3843
  arc A2 (-14.0462, 214.4522) -> (-20.3962, 220.8022) centre (-20.3962, 214.4522) ccw
  line L0 (-14.0462, 214.4522) -> (-14.0462, 1.7272)
  line L1 (-14.0462, 1.7272) -> (-26.7462, 1.7272)
  line L2 (-26.7462, 1.7272) -> (-26.7462, 220.8022)
  line L3 (-26.7462, 220.8022) -> (-20.3962, 220.8022)
  circle A3 centre (-20.3962, 34.1122) radius 1.905
  circle A4 centre (-20.3962, 195.4022) radius 1.905
  dimension "d191" = 3.81
  dimension "d192" = 3.81
  constraint concentric A1 A3
  constraint concentric A0 A4
  measures "d191" diameter of A3
  measures "d192" diameter of A4
extrude "Extrude27" cut sketch "Small Wall Thru Hole" against normal up to surface (5.2832 mm away) contours A0 | A1 | A3 | A4 bodies 13
extrude "Extrude28" cut sketch "Base" against normal up to surface (12.7 mm away) contours A16 | A17 | A18 | A19 bodies 1
sketch "Left Side Wall 1" plane through (0, 26.7462, 0) normal (0, -1, 0) x (1, 0, 0)
  arc A0 (648.7668, 214.4522) -> (642.4168, 220.8022) centre (642.4168, 214.4522) ccw
  line L0 (642.4168, 220.8022) -> (431.8508, 220.8022)
  line L1 (431.8508, 220.8022) -> (431.8508, -3.3528)
  line L2 (431.8508, -3.3528) -> (648.7668, -3.3528)
  line L3 (648.7668, -3.3528) -> (648.7668, 214.4522)
  circle A1 centre (642.4168, 195.4022) radius 1.905
  circle A2 centre (642.4168, 34.1122) radius 1.905
  dimension "d221" = 3.81
  dimension "d222" = 6.35
  dimension "d223" = 25.4
  dimension "d224" = 3.81
  dimension "d225" = 6.35
  dimension "d226" = 37.465
  measures "d221" diameter of A1
  measures "d222" distance of L3 A1.centre
  measures "d223" distance of L0 A1.centre
  measures "d224" diameter of A2
  measures "d225" distance of L3 A2.centre
  measures "d226" distance of L2 A2.centre
extrude "Extrude29" cut sketch "Left Side Wall 1" against normal up to surface (5.3086 mm away) contours A1 | A2 bodies 23
extrude "Extrude30" cut sketch "Small Wall Thru Hole" against normal up to surface (10.5918 mm away) contours A0 | A1 | A3 | A4 bodies 3
sketch "Left Side Wall 2" plane through (0, 26.7462, 0) normal (0, -1, 0) x (1, 0, 0)
  line L0 (426.5422, 220.8022) -> (236.1438, 220.8022)
  line L1 (236.1438, 220.8022) -> (236.1438, -3.3528)
  line L2 (236.1438, -3.3528) -> (426.5422, -3.3528)
  line L3 (426.5422, -3.3528) -> (426.5422, 220.8022)
sketch "Front Wall" plane through (636.0668, 0, 0) normal (1, 0, 0) x (0, 1, 0)
  line L0 (437.8452, -3.3528) -> (437.8452, 220.8022)
  line L1 (437.8452, 220.8022) -> (32.0548, 220.8022)
  line L2 (32.0548, 220.8022) -> (32.0548, -3.3528)
  line L3 (32.0548, -3.3528) -> (437.8452, -3.3528)
sketch "Front Left Inner Wall" plane through (431.8508, 0, 0) normal (1, 0, 0) x (0, 1, 0)
  circle A0 centre (20.3962, 195.4022) radius 1.905
  circle A1 centre (20.3962, 34.1122) radius 1.905
  arc A2 (20.3962, 220.8022) -> (14.0462, 214.4522) centre (20.3962, 214.4522) ccw
  line L0 (14.0462, 214.4522) -> (14.0462, -3.3528)
  line L1 (14.0462, -3.3528) -> (189.8215, -3.3528)
  line L2 (189.8215, -3.3528) -> (189.8215, 220.8022)
  line L3 (189.8215, 220.8022) -> (20.3962, 220.8022)
equation "d111 = 16 in + 2.2 in"
named bodies: "Base", "Front Right Inner Wall", "Front Left Inner Wall", "Rear Right Inner Wall", "Rear Left Inner Wall", "Rear Wall", "Front Wall", "Right Side Wall 1", "Left Side Wall 3", "Right Side Wall 2", "Left Side Wall 1", "Left Side Wall 2", "Right Side Wall 3", "Left Sled Arm", "Right Sled Arm", "Camera Beam"
